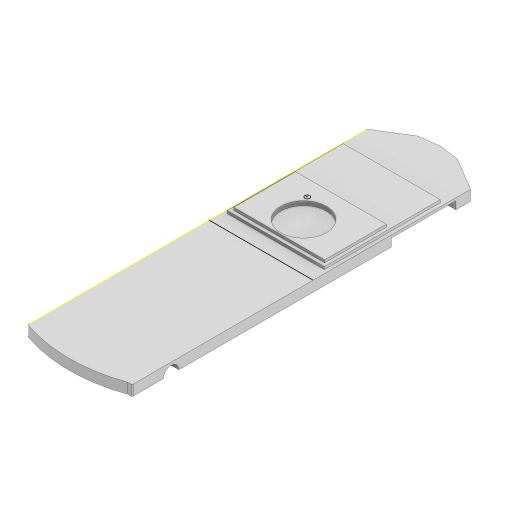
# Autodesk Inventor part: BASE
Saved by Autodesk Inventor 2024 (Build 280153000, 153)
## iProperties
Created: 2023-05-11
Part Number: BASE
Material: Generic
Document SubType Name: Modeling
Designer: Lenovo
Density: 1 g/cm^3
Appearance: Default
Author: Lenovo
Autodesk Inventor part; units mm, degrees
ref_plane "YZ Plane" through (0, 0, 0) normal (1, 0, 0) x (0, 1, 0)
ref_plane "XZ Plane" through (0, 0, 0) normal (0, 1, 0) x (-1, 0, 0)
ref_plane "XY Plane" through (0, 0, 0) normal (0, 0, 1) x (1, 0, 0)
sketch "Sketch1" plane through (0, 0, 0) normal (0, 1, 0) x (-1, 0, 0)
  line L0 (-100, 325) -> (100, 325)
  line L1 (100, 325) -> (100, -325)
  line L2 (100, -325) -> (-100, -325)
  line L3 (-100, -325) -> (-100, 325)
  line L4 (-100, 325) -> (100, -325) construction
  line L5 (100, 325) -> (-100, -325) construction
  point P0 (0, 0)
  dimension "d0" = 200
  dimension "d1" = 650
  constraints: 12 end point, 2 midpoint, 2 parallel, 1 horizontal, 1 perpendicular
  measures "d0" distance of L1.end L2.end
  measures "d1" distance of L0.end L1.end
sketch "Sketch2" plane through (0, 0, 0) normal (0, 1, 0) x (-1, 0, 0)
  point P0 (0, 0)
extrude "Extrusion1" add sketch "Sketch1" along normal blind 20
sketch "Sketch3" plane through (0, 20, 0) normal (0, 1, 0) x (1, 0, 0)
  line L0 (-100, -325) -> (100, -325) projected
  arc A0 (-100, -325) -> (91.7903, -325) centre (-4.1048, -57.5933) ccw
  point P0 (0, 0)
  constraints: 2 point on circle, 1 centre point, 1 point on line
extrude "Extrusion2" add sketch "Sketch3" against normal blind 20
sketch "Sketch4" plane through (0, 20, 0) normal (0, 1, 0) x (1, 0, 0)
  line L0 (100, 325) -> (-100, 325) projected
  line L1 (100, 325) -> (36.9346, 362.619)
  line L2 (36.9346, 362.619) -> (0, 367.9885)
  line L3 (0, 367.9885) -> (-39.4325, 362.619)
  line L4 (-39.4325, 362.619) -> (-100, 325)
  point P0 (0, 0)
  constraints: 8 end point
extrude "Extrusion3" add sketch "Sketch4" against normal blind 20
fillet "Fillet1" radius 2 1 edges at (100, 10, 325)
fillet "Fillet2" radius 4 1 edges at (-100, 10, 325)
chamfer "Chamfer1" distance 2 angle 45 1 edges at (0, 10, -367.9885)
fillet "Fillet3" radius 5 1 edges at (36.9346, 10, -362.619)
fillet "Fillet4" radius 5 1 edges at (-39.4325, 10, -362.619)
sketch "Sketch5" plane through (0, 20, 0) normal (0, 1, 0) x (1, 0, 0)
  line L0 (0, 22.7202) -> (-100, 22.7202)
  line L1 (-100, 325) -> (-100, -322.17) projected
  line L2 (0, 22.7202) -> (99.1127, 22.7202)
  line L3 (99.1127, 22.7202) -> (-100, 22.7202)
  point P0 (0, 0)
  constraints: 6 end point, 2 point on line, 1 horizontal, 1 perpendicular
sketch "Sketch6" plane through (0, 20, 0) normal (0, 1, 0) x (1, 0, 0)
  line L0 (93.1857, 273.63) -> (-93.1857, 273.63)
  line L1 (-93.1857, 273.63) -> (-93.1857, 51.0381)
  line L2 (-93.1857, 51.0381) -> (93.1857, 51.0381)
  line L3 (93.1857, 51.0381) -> (93.1857, 273.63)
  line L4 (93.1857, 273.63) -> (-93.1857, 51.0381) construction
  line L5 (-93.1857, 273.63) -> (93.1857, 51.0381) construction
  point P0 (0, 0)
  point P1 (0, 162.334)
  constraints: 12 end point, 2 midpoint, 2 parallel, 1 horizontal, 1 perpendicular
extrude "Extrusion4" add sketch "Sketch6" along normal blind 5
sketch "Sketch7" plane through (0, 25, 0) normal (0, 1, 0) x (1, 0, 0)
  line L0 (87.2587, 176.1637) -> (-87.2587, 176.1637)
  line L1 (-87.2587, 176.1637) -> (-87.2587, 57.6236)
  line L2 (-87.2587, 57.6236) -> (87.2587, 57.6236)
  line L3 (87.2587, 57.6236) -> (87.2587, 176.1637)
  line L4 (87.2587, 176.1637) -> (-87.2587, 57.6236) construction
  line L5 (-87.2587, 176.1637) -> (87.2587, 57.6236) construction
  point P0 (0, 0)
  point P1 (0, 116.8937)
  constraints: 12 end point, 2 midpoint, 2 parallel, 1 horizontal, 1 perpendicular
extrude "Extrusion5" add sketch "Sketch7" along normal blind 5
sketch "Sketch8" plane through (0, 30, 0) normal (0, 1, 0) x (1, 0, 0)
  circle A0 centre (0, 104.3811) radius 44.0999
  point P0 (0, 0)
  constraints: 1 centre point
extrude "Extrusion6" cut sketch "Sketch8" against normal blind 8
sketch "Sketch9" plane through (0, 30, 0) normal (0, 1, 0) x (1, 0, 0)
  circle A0 centre (-34.3381, 145.486) radius 4.7269
  point P0 (0, 0)
  constraints: 1 centre point
sketch "Sketch10" plane through (0, 0, 0) normal (0, -1, 0) x (1, 0, 0)
  line L0 (100, 323) -> (100, -325) projected
  line L1 (100, -296.7409) -> (61.6936, -296.7409)
  line L2 (61.6936, -296.7409) -> (61.6936, -172.3341)
  line L3 (61.6936, -172.3341) -> (100, -172.3341)
  line L4 (100, -172.3341) -> (100, -296.7409)
  point P0 (0, 0)
  constraints: 8 end point, 2 parallel, 1 horizontal, 1 perpendicular, 1 point on line
extrude "Extrusion7" cut sketch "Sketch10" against normal blind 15
sketch "Sketch11" plane through (0, 0, 0) normal (0, -1, 0) x (1, 0, 0)
  line L0 (-100, -325) -> (-100, 322.17) projected
  line L1 (-87.2587, -176.1637) -> (87.2587, -176.1637) projected
  line L2 (-100, -294.7015) -> (-69.8514, -294.7015)
  line L3 (-69.8514, -294.7015) -> (-69.8514, -176.1637)
  line L4 (-69.8514, -176.1637) -> (-100, -176.1637)
  line L5 (-100, -176.1637) -> (-100, -294.7015)
  point P0 (0, 0)
  constraints: 8 end point, 2 parallel, 2 point on line, 1 horizontal, 1 perpendicular
extrude "Extrusion8" cut sketch "Sketch11" against normal blind 15
sketch "Sketch12" plane through (100, 0, -325) normal (1, 0, 0) x (0, 0, -1)
  circle A0 centre (-575.0278, 0) radius 14.8623
  point P0 (-325, 0)
  constraints: 1 centre point
extrude "Extrusion9" cut sketch "Sketch12" against normal blind 15
sketch "Sketch13" plane through (-100, 0, -325) normal (-1, 0, 0) x (0, 0, 1)
  line L0 (560.1655, 0) -> (589.8902, 0) projected
  circle A0 centre (575.0278, 0) radius 14.8623
  point P0 (325, 0)
  constraints: 1 centre point, 1 midpoint
extrude "Extrusion10" cut sketch "Sketch13" against normal blind 15
body "Solid1"
